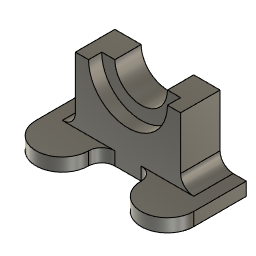
NCV-17 v2 (Autodesk Fusion 360 design; units mm, degrees)
Autodesk Fusion 360 part; units mm, degrees
note: some values were not read from the file. Set by a fixed rule: which sketch regions a step uses.
sketch "Sketch1" plane through (0, 0, 0) normal (0, 1, 0) x (1, 0, 0)
  line L0 (0, 0) -> (60, 0)
  line L1 (60, 0) -> (60, -10)
  line L2 (60, -10) -> (50, -10)
  line L3 (40, -20) -> (40, -60)
  line L4 (-40, -60) -> (-40, -20)
  line L5 (-50, -10) -> (-60, -10)
  line L6 (-60, -10) -> (-60, 0)
  line L7 (-60, 0) -> (0, 0)
  arc A0 (-40, -20) -> (-50, -10) centre (-50, -20) ccw
  arc A1 (50, -10) -> (40, -20) centre (50, -20) ccw
  arc A2 (20, -60) -> (-20, -60) centre (0, -60) ccw
  arc A3 (30, -60) -> (-30, -60) centre (0, -60) ccw
  line L8 (40, -60) -> (20, -60)
  line L9 (-20, -60) -> (-40, -60)
  dimension "d1" = 60
  dimension "d2" = 60
  dimension "d3" = 10
  dimension "d4" = 10
  dimension "d5" = 10
  dimension "d6" = 40
  dimension "d7" = 40
  dimension "d8" = 60
  dimension "d9" = 40
  dimension "d10" = 40
  dimension "d11" = 60
  dimension "d12" = 40
  constraint coincident L0.start L7.end
  constraint horizontal L0
  constraint parallel L0 L2
  constraint parallel L0 L8
  constraint perpendicular L4 L8
  constraint parallel L0 L7
  constraint vertical L1
  constraint vertical L6
  constraint horizontal L5
  constraint vertical L3
  constraint tangent L4 A0
  constraint tangent L5 A0
  constraint tangent L2 A1
  constraint tangent L3 A1
  constraint equal A0 A1
  constraint coincident A2.centre L8
  constraint coincident A2.end L8
  constraint coincident A3.end L8
  constraint coincident A3.start L8
  constraint collinear L8 L9
  measures "d1" distance of L0.start L0.end
  measures "d2" distance of L0.start L6.end
  measures "d3" radius of A0
  measures "d4" vertical distance of L0.start L5.end
  measures "d5" distance of L0.end L1.end
  measures "d6" horizontal distance of L0.start L3.start
  measures "d7" horizontal distance of L0.start L4.end
  measures "d8" distance of L0.start L8
  measures "d9" distance of L3 A2.centre
  measures "d10" diameter of A2
  measures "d11" diameter of A3
  measures "d12" distance of L3 A2.centre
sketch "Sketch2" plane through (0, 0, 0) normal (0, 0, 1) x (1, 0, 0)
  line L0 (60, 0) -> (60, -40)
  line L1 (0, 0) -> (0, -30)
  line L2 (0, -30) -> (10, -30)
  arc A0 (20, -40) -> (60, -40) centre (40, -40) ccw
  line L3 (0, 0) -> (60, 0)
  arc A1 (20, -40) -> (10, -30) centre (10, -40) ccw
  dimension "d18" = 60
  dimension "d21" = 60
  dimension "d22" = 30
  dimension "d23" = 40
  dimension "d24" = 40
  dimension "d26" = 40
  dimension "d27" = 40
  dimension "d28" = 10
  dimension "d33" = 20
  constraint vertical L0
  constraint coincident L1.start L3.start
  constraint horizontal L2
  constraint horizontal L3
  constraint tangent L2 A1
  constraint tangent A0 A1
  measures "d18" distance of L0 L1.start
  measures "d21" distance of L0 L1
  measures "d22" distance of L1.start L2
  measures "d23" diameter of A0
  measures "d24" horizontal distance of L1.start A0.centre
  measures "d26" vertical distance of L0.end L1.start
  measures "d27" vertical distance of L1.start A0.start
  measures "d28" horizontal distance of L1.start L2.end
  measures "d33" diameter of A1
extrude "Extrude1" add sketch "Sketch1" against normal blind 30 contours L0 L1 L2 L3 L4 L5 L6 L7 A0 A1 A3 L8 L9
extrude "Extrude2" add sketch "Sketch1" against normal blind 20 contours A2 A3 L8 L9
extrude "Extrude3" add sketch "Sketch2" along normal blind 10
mirror "Mirror1" about plane through (0, 0, 0) normal (1, 0, 0) of "Extrude3"
equation "d9 = d6"
equation "d12 = d6"
